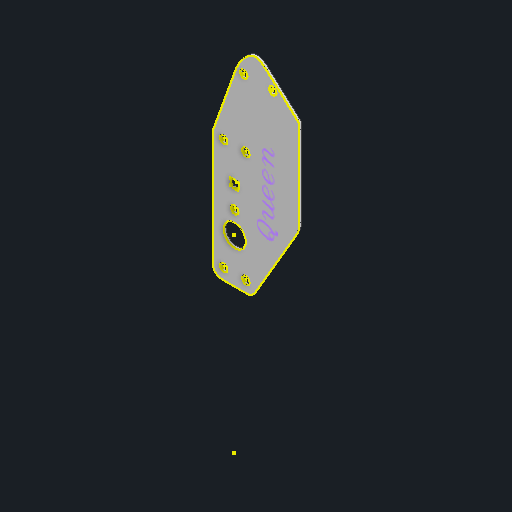
# Autodesk Inventor part: sled
Saved by Autodesk Inventor 2024 (Build 280153000, 153)
## iProperties
Created: 2023-04-17
Part Number: sled
Material: Generic
Document SubType Name: Modeling
Designer: Liam
Density: 1 g/cm^3
Appearance: Default
Author: Liam
Autodesk Inventor part; units mm, degrees
ref_plane "YZ Plane" through (0, 0, 0) normal (1, 0, 0) x (0, 1, 0)
ref_plane "XZ Plane" through (0, 0, 0) normal (0, 1, 0) x (-1, 0, 0)
ref_plane "XY Plane" through (0, 0, 0) normal (0, 0, 1) x (1, 0, 0)
sketch "Sketch1" plane through (0, 0, 0) normal (0, 0, 1) x (1, 0, 0)
  circle A0 centre (-6.35, 152.4) radius 2.1844
  circle A1 centre (6.35, 152.4) radius 2.1844
  circle A2 centre (-6.35, 88.9) radius 2.1844
  circle A3 centre (6.35, 88.9) radius 2.1844
  arc A4 (-1.8034, 135.6614) -> (-2.3114, 135.1534) centre (-1.8034, 135.1534) ccw
  line L0 (-2.3114, 131.5466) -> (-2.3114, 135.1534)
  line L1 (-1.8034, 135.6614) -> (1.8034, 135.6614)
  arc A5 (-2.3114, 131.5466) -> (-1.8034, 131.0386) centre (-1.8034, 131.5466) ccw
  line L2 (1.8034, 131.0386) -> (-1.8034, 131.0386)
  arc A6 (1.8034, 131.0386) -> (2.3114, 131.5466) centre (1.8034, 131.5466) ccw
  line L3 (2.3114, 135.1534) -> (2.3114, 131.5466)
  arc A7 (2.3114, 135.1534) -> (1.8034, 135.6614) centre (1.8034, 135.1534) ccw
  circle A8 centre (0, 120.65) radius 2.1844
  circle A9 centre (0, 107.95) radius 6.35
  line L4 (36.7693, 131.7499) -> (36.7693, 177.9954)
  line L5 (-12.7, 88.9) -> (-12.7, 152.4)
  line L6 (-6.35, 82.55) -> (6.35, 82.55)
  spline S0 degree 4 poles (-12.7, 88.9) (-12.7, 87.6131) (-12.7, 85.0392) (-10.2108, 82.55) (-7.6369, 82.55) (-6.35, 82.55) knots 0 0 0 0 0 0.5 1 1 1 1 1
  spline S1 degree 4 poles (6.35, 82.55) (8.1081, 82.55) (9.8661, 82.55) (11.0889, 84.4373) (11.9675, 85.9392) knots 0 0 0 0 0 1 1 1 1 1
  line L7 (11.9675, 85.9392) -> (33.5511, 122.8344)
  spline S2 degree 4 poles (33.5511, 122.8344) (34.1544, 123.8656) (35.3609, 125.928) (36.7693, 128.0899) (36.7693, 130.5299) (36.7693, 131.7499) knots 0 0 0 0 0 0.5 1 1 1 1 1
  spline S3 degree 4 poles (-11.9358, 155.4201) (-12.0668, 155.0524) (-12.3287, 154.3171) (-12.7, 153.5861) (-12.7, 152.7954) (-12.7, 152.4) knots 0 0 0 0 0 0.5 1 1 1 1 1
  line L8 (-11.9358, 155.4201) -> (0, 188.9294)
  line L9 (18.2111, 198.8461) -> (35.8036, 182.8241)
  spline S4 degree 4 poles (0, 188.9294) (0.9805, 191.6822) (2.9416, 197.1879) (10.5283, 205.8431) (15.6502, 201.1784) (18.2111, 198.8461) knots 0 0 0 0 0 0.5 1 1 1 1 1
  spline S5 degree 4 poles (35.8036, 182.8241) (36.303, 182.3693) (37.3018, 181.4596) (36.7693, 179.86) (36.7693, 178.6169) (36.7693, 177.9954) knots 0 0 0 0 0 0.5 1 1 1 1 1
  circle A10 centre (21.7424, 190.5) radius 2.1844
  circle A11 centre (5.1816, 190.5) radius 2.1844
  point P0 (0, 0)
  point P1 (21.7424, 177.8)
  point P2 (14.224, 190.5)
  dimension "d1" = 4.3688
  dimension "d2" = 12.7
  dimension "d10" = 0
  dimension "d13" = 16.5608
  dimension "d16" = 12.7
  dimension "d17" = 7.5184
  constraints: 20 end point, 12 centre point, 8 point on circle, 7 vertical, 6 equal radius, 4 horizontal, 30 other
  measures "d1" diameter of A0
  measures "d2" diameter of A9
  measures "d10" vertical distance of A10.centre A11.centre
  measures "d13" distance of A10.centre A11.centre
  measures "d16" distance of A10.centre point (21.742, 177.8)
  measures "d17" distance of A10.centre point (14.224, 190.5)
extrude "Extrusion1" add sketch "Sketch1" along normal blind 1.524
sketch "Sketch2" plane through (0, 0, 1.524) normal (0, 0, 1) x (1, 0, 0)
  line L0 (12.9318, 114.6329) -> (12.9318, 139.693) construction
  line L1 (12.9318, 139.693) -> (20.9407, 139.693) construction
  line L2 (20.9407, 139.693) -> (20.9407, 114.6329) construction
  line L3 (20.9407, 114.6329) -> (12.9318, 114.6329) construction
  line L4 (-6.35, 82.55) -> (6.35, 82.55) projected
  line L5 (11.9675, 85.9392) -> (33.5511, 122.8344) projected
  line L6 (36.7693, 131.7499) -> (36.7693, 177.9954) projected
  line L7 (35.8036, 182.8241) -> (18.2111, 198.8461) projected
  line L8 (0, 188.9294) -> (-11.9358, 155.4201) projected
  line L9 (-12.7, 152.4) -> (-12.7, 88.9) projected
  circle A0 centre (-6.35, 152.4) radius 2.1844 projected
  circle A1 centre (6.35, 152.4) radius 2.1844 projected
  circle A2 centre (6.35, 88.9) radius 2.1844 projected
  circle A3 centre (0, 120.65) radius 2.1844 projected
  circle A4 centre (0, 107.95) radius 6.35 projected
  circle A5 centre (21.7424, 190.5) radius 2.1844 projected
  circle A6 centre (5.1816, 190.5) radius 2.1844 projected
  line L10 (2.3114, 135.1534) -> (2.3114, 131.5466) projected
  arc A7 (1.8034, 131.0386) -> (2.3114, 131.5466) centre (1.8034, 131.5466) ccw projected
  line L11 (1.8034, 131.0386) -> (-1.8034, 131.0386) projected
  arc A8 (-2.3114, 131.5466) -> (-1.8034, 131.0386) centre (-1.8034, 131.5466) ccw projected
  line L12 (-2.3114, 131.5466) -> (-2.3114, 135.1534) projected
  arc A9 (-1.8034, 135.6614) -> (-2.3114, 135.1534) centre (-1.8034, 135.1534) ccw projected
  line L13 (-1.8034, 135.6614) -> (1.8034, 135.6614) projected
  arc A10 (2.3114, 135.1534) -> (1.8034, 135.6614) centre (1.8034, 135.1534) ccw projected
  circle A11 centre (-6.35, 88.9) radius 2.1844 projected
  point P0 (0, 0)
  constraints: 8 other
body "Solid1"
